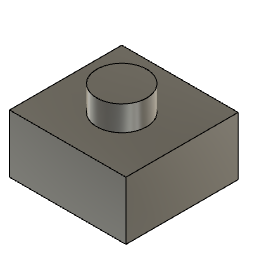
LEDClamp (Autodesk Fusion 360 design; units mm, degrees)
Autodesk Fusion 360 part; units mm, degrees
note: some values were not read from the file. Chosen so that the rebuilt part matches the saved one: that a step has no effect.
sketch "Skizze32" plane through (0, 0, 0) normal (0, 0, 1) x (1, 0, 0)
  line L0 (42, 7) -> (28, 7)
  line L1 (28, 7) -> (28, -6.5)
  line L2 (28, -6.5) -> (42, -6.5)
  line L3 (42, -6.5) -> (42, 7)
  line L4 (42, 7) -> (28, -6.5) construction
  line L5 (28, 7) -> (42, -6.5) construction
  point P0 (35, 0.25)
  dimension "d217" = 14
  dimension "d218" = 13.5
  constraint horizontal L0
  constraint perpendicular L0 L1
  constraint parallel L0 L2
  constraint parallel L1 L3
  constraint coincident L4 P0
  constraint coincident L5 P0
  measures "d217" distance of L1.end L2.end
  measures "d218" distance of L0.end L1.end
extrude "Extrusion36" add sketch "Skizze32" along normal blind 7
sketch "Skizze34" plane through (0, 0, 7) normal (0, 0, 1) x (-1, 0, 0)
  line L0 (-42, 6.5) -> (-42, -7)
  line L1 (-42, -7) -> (-28, -7)
  line L2 (-28, -7) -> (-28, 6.5)
  line L3 (-28, 6.5) -> (-42, 6.5)
  circle A0 centre (-35, 0) radius 3
  dimension "d223" = 6
  measures "d223" diameter of A0
extrude "Extrusion37" add sketch "Skizze34" along normal blind 3 contours A0
sketch "Skizze35" plane through (0, 7, 0) normal (0, 1, 0) x (-1, 0, 0)
  line L0 (-42, 0) -> (-28, 0)
  line L1 (-28, 0) -> (-28, 7)
  line L2 (-28, 7) -> (-42, 7)
  line L3 (-42, 7) -> (-42, 0)
  line L4 (-36.5, 6) -> (-33.5, 6)
  line L5 (-33.5, 6) -> (-33.5, 0)
  line L6 (-33.5, 0) -> (-36.5, 0)
  line L7 (-36.5, 0) -> (-36.5, 6)
  constraint horizontal L4
  constraint vertical L5
  constraint horizontal L6
  constraint vertical L7
  constraint coincident L0 L5.end
extrude "Extrusion38" add sketch "Skizze35" along normal blind 1 contours L0 L4 L5 L6 L7
fillet "Abrundung3" radius 0.3 3 edges at (33.5, 8, 3) (36.5, 8, 3) (35, 8, 6)
extrude "Extrusion39" [no effect]
